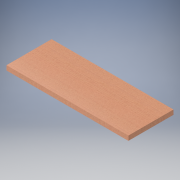
# Autodesk Inventor part: Deck
Saved by Autodesk Inventor 2019 (Build 230136000, 136)
## iProperties
Created: 2020-12-25
Part Number: Deck
Material: Wood (Oak)
Document SubType Name: Modeling
Designer: John
Density: 0.76 g/cm^3
Appearance: White Oak - Natural Medium Gloss
Author: John
Autodesk Inventor part; units mm, degrees
ref_plane "YZ Plane" through (0, 0, 0) normal (1, 0, 0) x (0, 1, 0)
ref_plane "XZ Plane" through (0, 0, 0) normal (0, 1, 0) x (-1, 0, 0)
ref_plane "XY Plane" through (0, 0, 0) normal (0, 0, 1) x (1, 0, 0)
sketch "Sketch1" plane through (0, 0, 0) normal (0, 1, 0) x (-1, 0, 0)
  line L0 (-454, 168) -> (454, 168)
  line L1 (454, 168) -> (454, -168)
  line L2 (454, -168) -> (-454, -168)
  line L3 (-454, -168) -> (-454, 168)
  line L4 (-454, 168) -> (454, -168) construction
  line L5 (454, 168) -> (-454, -168) construction
  point P0 (0, 0)
  dimension "d0" = 908
  dimension "d1" = 336
  constraints: 12 end point, 2 midpoint, 2 parallel, 1 horizontal, 1 perpendicular
  measures "d0" distance of L1.end L2.end
  measures "d1" distance of L0.end L1.end
extrude "Extrusion1" add sketch "Sketch1" along normal blind 34.29
body "Solid1"
